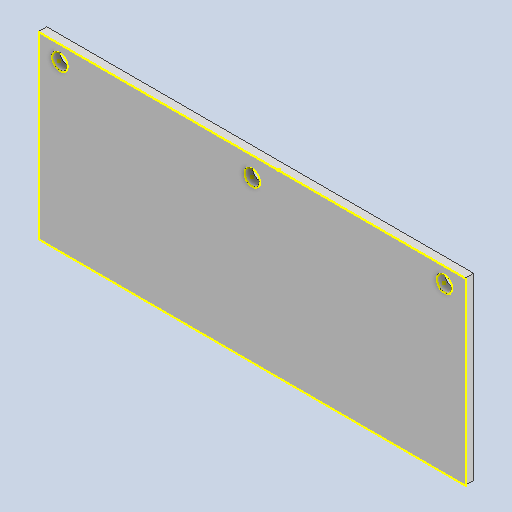
# Autodesk Inventor part: PCBE_2_2
Saved by Autodesk Inventor 2023 (Build 270158000, 158)
## iProperties
Created: 2023-04-06
Part Number: PCBE_2_2
Material: Ogólny
Document SubType Name: Modeling
Designer: Kamil
Density: 1 g/cm^3
Appearance: Domyślna
Author: Kamil
Autodesk Inventor part; units mm, degrees
ref_plane "YZ Plane" through (0, 0, 0) normal (1, 0, 0) x (0, 1, 0)
ref_plane "XZ Plane" through (0, 0, 0) normal (0, 1, 0) x (-1, 0, 0)
ref_plane "XY Plane" through (0, 0, 0) normal (0, 0, 1) x (1, 0, 0)
sketch "Szkic1" plane through (0, 0, 0) normal (0, 0, 1) x (1, 0, 0)
  circle A0 centre (-5.2, -2.45) radius 1.5 projected
  line L0 (-10.4, 2.5) -> (0, 2.5) projected
  line L1 (-10.4, 2.5) -> (-10.4, -7.4) projected
  line L2 (-10.4, -7.4) -> (0, -7.4) projected
  line L3 (0, 2.5) -> (0, -7.4) projected
  line L4 (-47.2, 2.5) -> (36.8, 2.5) projected
  line L5 (-47.2, -36.8743) -> (-47.2, 14.8735) projected
  line L6 (36.8, -36.8743) -> (36.8, 14.8735) projected
  line L7 (-47.2, 2.5) -> (36.8, 2.5)
  line L8 (36.8, 2.5) -> (36.8, -36.8743)
  line L9 (36.8, -36.8743) -> (-47.2, -36.8743)
  line L10 (-47.2, -36.8743) -> (-47.2, 2.5)
  line L11 (-44.7, -34.3743) -> (34.3, -34.3743)
  line L12 (34.3, -34.3743) -> (34.3, 0)
  line L13 (34.3, 0) -> (-44.7, 0)
  line L14 (-44.7, 0) -> (-44.7, -34.3743)
  line L15 (-5.2, 0) -> (-5.2, -7.4)
  circle A1 centre (-5.2, -3.7) radius 1.5
  point P0 (0, 0)
  dimension "d0" = 2.5
  constraints: 18 end point, 4 parallel, 3 midpoint, 2 perpendicular, 1 centre point, 1 horizontal, 3 other
  measures "d0" distance between parallel lines of L9 L11
extrude "Wyciągnięcie proste1" add sketch "Szkic1" along normal blind 1.6 contours A0 A1 L15 | A0 L15 L13 L3 L2 A1 | L15 A1 A0 | A0 A1 L15 L2 L1 L13 | L13 L12 L11 L14 L1 L2 L3 picked at (-4.9756, -1.8088) picked at (-5.4233, -1.8086)
sketch "Szkic2" plane through (0, 0, 1.6) normal (0, 0, 1) x (1, 0, 0)
  circle A0 centre (-42.05, -2.9) radius 1.5 projected
  circle A1 centre (31.65, -2.9) radius 1.5 projected
  point P0 (0, 0)
extrude "Wyciągnięcie proste2" cut sketch "Szkic2" against normal through all
sketch "Szkic3" plane through (0, 0, 1.6) normal (0, 0, 1) x (1, 0, 0)
  circle A0 centre (31.65, -2.9) radius 1.5 projected
  circle A1 centre (-42.05, -2.9) radius 1.5 projected
  line L0 (-44.7, 0) -> (-44.7, -34.3743) projected
  line L1 (-44.7, -34.3743) -> (34.3, -34.3743) projected
  line L2 (34.3, -34.3743) -> (34.3, 0) projected
  line L3 (34.3, 0) -> (-44.7, 0) projected
  circle A2 centre (-5.2, -3.7) radius 1.5 projected
  line L4 (-44.7, 0) -> (-44.7, -34.3743) projected
  line L5 (34.3, 0) -> (-44.7, 0) projected
  line L6 (-44.7, -34.3743) -> (34.3, -34.3743)
  line L7 (34.3, -34.3743) -> (34.3, 0)
  line L8 (34.3, 0) -> (-44.7, 0)
  line L9 (-44.7, 0) -> (-44.7, -34.3743)
  line L10 (-46.1, 0) -> (-46.1, -34.3743)
  line L11 (35.7, 0) -> (35.7, -35.7743)
  line L12 (35.7, -35.7743) -> (-44.7, -35.7743)
  line L13 (-46.1, -34.3743) -> (35.7, -34.3743)
  line L14 (-44.7, -34.3743) -> (34.3, -34.3743) projected
  line L15 (-46.1, 0) -> (35.7, 0)
  point P0 (0, 0)
  dimension "d5" = 1.4
  dimension "d6" = 1.4
  constraints: 18 end point, 3 parallel, 2 collinear, 1 horizontal, 1 perpendicular, 1 point on line, 1 other
  measures "d5" distance between parallel lines of L0 L10
  measures "d6" distance between parallel lines of L2 L11
extrude "Wyciągnięcie proste3" add sketch "Szkic3" against normal up to surface (1.6 mm away) contours L0 L13 L10 L15 | L15 L11 L13 L2
sketch "Szkic5" plane through (0, 0, 1.6) normal (0, 0, 1) x (1, 0, 0)
  circle A0 centre (31.65, -2.9) radius 1.5 projected
  circle A1 centre (-42.05, -2.9) radius 1.5 projected
  line L0 (-46.1, -34.3743) -> (35.7, -34.3743) projected
  line L1 (35.7, -34.3743) -> (35.7, 0) projected
  line L2 (35.7, 0) -> (-46.1, 0) projected
  line L3 (-46.1, 0) -> (-46.1, -34.3743) projected
  circle A2 centre (-5.2, -3.7) radius 1.5 projected
  point P0 (0, 0)
